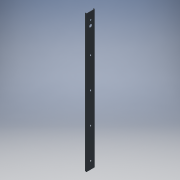
# Autodesk Inventor part: rail_SSRN3618
Saved by Autodesk Inventor 2016 (Build 200138000, 138)
## iProperties
Category: PARTsolutions
Company: MISUMI
Created: 2016-11-23
Part Number: rail_SSRN3618
Catalog Web Link: www.cadenas.de
Description: rail_ssrn36-Slide Rails - Stainles Steel - Two - Step Slide Rails
Vendor: MISUMI
Document SubType Name: Modeling
Designer: psAdmin
Manufacturer: MISUMI
Mass: 117.124 g
Surface Area: 322.81 cm^2
Volume: 16.381 cm^3
Density: 7.15 g/cm^3
Material: 鉄 灰色
Appearance: 鉄 灰色
PSOL_IDENT_0: {$CADENAS_DATA\23d-libs\misumi\metric\07_slide_rails\ssrn36_series\ssrn36_rail.prj},166 {VTYP=3D},{N
PSOL_IDENT_1: B=rail_SSRN3618},{LINA=rail_SSRN3618},{NN=rail_ssrn36},{DATE=17.06.2016 05:46:12},{GEOMDATE=16.03.20
PSOL_IDENT_2: 05},{VERSION=},{LINEID=10},{LINESUBID=-1},{WBVAR=NO}  {NB=rail_SSRN3618},{LINA=rail_SSRN3618},{KT=DU
PSOL_IDENT_3: MMY},{PN=SSRN3618},{TYPE=SSRN3618},{MATR=Rail 304 Stainless Steel},{MATB=Ball 440C Stainless Steel},
PSOL_IDENT_4: {NO=18},{RL=457.2},{TD=330.2},{A=203.2},{B=304.8},{C=406.4},{D=212.7},{E=301.6},{F=412.7},{G=425.4},
PSOL_IDENT_5: {RLD=402}
NN: rail_ssrn36
NT: Slide Rails - Stainles Steel - Two - Step Slide Rails
NB: rail_SSRN3618
NBSYN: rail_$PN.
LINA: rail_SSRN3618
MATR: Rail 304 Stainless Steel
MATB: Ball 440C Stainless Steel
NO: 18
SUPPLIER: MISUMI
ARTICLENO: rail_SSRN3618
BOMINFO: rail_SSRN3618
CREATOR: CADENAS GmbH
Title: rail_SSRN3618
Author: Cadenas PARTsolutions
Comments: Slide Rails - Stainles Steel - Two - Step Slide Rails
Autodesk Inventor part; units mm, degrees
sketch "Sketch_1" plane through (0, 0, 0) normal (0, 0, 1) x (1, 0, 0)
  arc A0 (1.8281, 29.2788) -> (4.2342, 27.8447) centre (3.65, 29.6) ccw
  arc A1 (5.55, 26.8958) -> (4.2342, 27.8447) centre (4.55, 26.8958) ccw
  line L0 (5.55, 26.8958) -> (5.55, 3.7042)
  arc A2 (4.2342, 2.7553) -> (5.55, 3.7042) centre (4.55, 3.7042) ccw
  arc A3 (4.2342, 2.7553) -> (1.8281, 1.3212) centre (3.65, 1) ccw
  line L1 (1.8281, 1.3212) -> (2.2787, 1.2418)
  arc A4 (4.8691, 1.3916) -> (2.2787, 1.2418) centre (3.65, 0) ccw
  arc A5 (4.8691, 1.3916) -> (6.3379, 1.5571) centre (5.528, 2.1437) ccw
  line L2 (6.3379, 1.5571) -> (6.55, 1.85)
  line L3 (6.55, 1.85) -> (6.55, 28.75)
  line L4 (6.55, 28.75) -> (6.3379, 29.0429)
  arc A6 (6.3379, 29.0429) -> (4.8691, 29.2084) centre (5.528, 28.4563) ccw
  arc A7 (2.2787, 29.3582) -> (4.8691, 29.2084) centre (3.65, 30.6) ccw
  line L5 (2.2787, 29.3582) -> (1.8281, 29.2788)
  constraints: 16 point on circle, 12 end point, 8 centre point
extrude "Extrusion1" add sketch "Sketch_1" along normal blind 457.2
sketch "Sketch2" plane through (6.55, 1.85, 0) normal (1, 0, 0) x (0, 0, -1)
  point P0 (-415.2, 13.45)
hole "Hole1" at (6.55, 15.3, 415.2) direction (-1, 0, 0) diameter 9.5 depth 1
sketch "Sketch_5" plane through (6.55, 0, 0) normal (1, 0, 0) x (0, 0, -1)
  line L0 (-434.05, 15.7) -> (-434.05, 14.9)
  arc A0 (-434.05, 14.9) -> (-431.8, 12.65) centre (-431.8, 14.9) ccw
  arc A1 (-431.8, 12.65) -> (-429.55, 14.9) centre (-431.8, 14.9) ccw
  line L1 (-429.55, 14.9) -> (-429.55, 15.7)
  arc A2 (-429.55, 15.7) -> (-431.8, 17.95) centre (-431.8, 15.7) ccw
  arc A3 (-431.8, 17.95) -> (-434.05, 15.7) centre (-431.8, 15.7) ccw
  constraints: 8 point on circle, 4 centre point, 4 end point
extrude "Extrusion2" cut sketch "Sketch_5" against normal blind 1
sketch "Sketch_6" plane through (6.55, 0, 0) normal (1, 0, 0) x (0, 0, -1)
  line L0 (-27.65, 15.7) -> (-27.65, 14.9)
  arc A0 (-27.65, 14.9) -> (-25.4, 12.65) centre (-25.4, 14.9) ccw
  arc A1 (-25.4, 12.65) -> (-23.15, 14.9) centre (-25.4, 14.9) ccw
  line L1 (-23.15, 14.9) -> (-23.15, 15.7)
  arc A2 (-23.15, 15.7) -> (-25.4, 17.95) centre (-25.4, 15.7) ccw
  arc A3 (-25.4, 17.95) -> (-27.65, 15.7) centre (-25.4, 15.7) ccw
  constraints: 8 point on circle, 4 centre point, 4 end point
extrude "Extrusion3" cut sketch "Sketch_6" against normal blind 1
sketch "Sketch_7" plane through (6.55, 0, 0) normal (1, 0, 0) x (0, 0, -1)
  arc A0 (-332.85, 15.3) -> (-330.6, 13.05) centre (-330.6, 15.3) ccw
  line L0 (-330.6, 13.05) -> (-329.8, 13.05)
  arc A1 (-329.8, 13.05) -> (-327.55, 15.3) centre (-329.8, 15.3) ccw
  arc A2 (-327.55, 15.3) -> (-329.8, 17.55) centre (-329.8, 15.3) ccw
  line L1 (-329.8, 17.55) -> (-330.6, 17.55)
  arc A3 (-330.6, 17.55) -> (-332.85, 15.3) centre (-330.6, 15.3) ccw
  constraints: 8 point on circle, 4 centre point, 4 end point
extrude "Extrusion4" cut sketch "Sketch_7" against normal blind 1
sketch "Sketch_8" plane through (6.55, 0, 0) normal (1, 0, 0) x (0, 0, -1)
  arc A0 (-231.25, 15.3) -> (-229, 13.05) centre (-229, 15.3) ccw
  line L0 (-229, 13.05) -> (-228.2, 13.05)
  arc A1 (-228.2, 13.05) -> (-225.95, 15.3) centre (-228.2, 15.3) ccw
  arc A2 (-225.95, 15.3) -> (-228.2, 17.55) centre (-228.2, 15.3) ccw
  line L1 (-228.2, 17.55) -> (-229, 17.55)
  arc A3 (-229, 17.55) -> (-231.25, 15.3) centre (-229, 15.3) ccw
  constraints: 8 point on circle, 4 centre point, 4 end point
extrude "Extrusion5" cut sketch "Sketch_8" against normal blind 1
sketch "Sketch_9" plane through (6.55, 0, 0) normal (1, 0, 0) x (0, 0, -1)
  arc A0 (-129.65, 15.3) -> (-127.4, 13.05) centre (-127.4, 15.3) ccw
  line L0 (-127.4, 13.05) -> (-126.6, 13.05)
  arc A1 (-126.6, 13.05) -> (-124.35, 15.3) centre (-126.6, 15.3) ccw
  arc A2 (-124.35, 15.3) -> (-126.6, 17.55) centre (-126.6, 15.3) ccw
  line L1 (-126.6, 17.55) -> (-127.4, 17.55)
  arc A3 (-127.4, 17.55) -> (-129.65, 15.3) centre (-127.4, 15.3) ccw
  constraints: 8 point on circle, 4 centre point, 4 end point
extrude "Extrusion6" cut sketch "Sketch_9" against normal blind 1
ref_plane "to_body_XY" through (6.5, 15.3, 228.6) normal (0, 0, 1) x (1, 0, 0)
ref_plane "to_body_YZ" through (6.5, 15.3, 228.6) normal (1, 0, 0) x (0, 1, 0)
ref_plane "to_body_ZX" through (6.5, 15.3, 228.6) normal (0, 1, 0) x (0, 0, 1)
ref_plane "to_slider_XY" through (6.5, 15.3, 228.6) normal (0, 0, 1) x (1, 0, 0)
ref_plane "to_slider_YZ" through (6.5, 15.3, 228.6) normal (1, 0, 0) x (0, 1, 0)
ref_plane "to_slider_ZX" through (6.5, 15.3, 228.6) normal (0, 1, 0) x (0, 0, 1)
body "Solid1"
